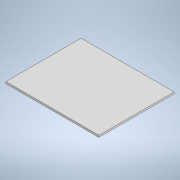
# Autodesk Inventor part: False_Bottom
Saved by Autodesk Inventor 2020 (Build 240168000, 168)
## iProperties
Created: 2021-12-09
Part Number: False_Bottom
Material: Generic
Document SubType Name: Modeling
Designer: danie
Density: 1 g/cm^3
Appearance: Default
Author: danie
Autodesk Inventor part; units mm, degrees
ref_plane "YZ Plane" through (0, 0, 0) normal (1, 0, 0) x (0, 1, 0)
ref_plane "XZ Plane" through (0, 0, 0) normal (0, 1, 0) x (-1, 0, 0)
ref_plane "XY Plane" through (0, 0, 0) normal (0, 0, 1) x (1, 0, 0)
sketch "Sketch1" plane through (0, 0, 0) normal (0, 1, 0) x (-1, 0, 0)
  line L0 (0, 0) -> (-155.575, 0)
  line L1 (-155.575, 0) -> (-155.575, 125.73)
  line L2 (-155.575, 125.73) -> (0, 125.73)
  line L3 (0, 125.73) -> (0, 0)
  dimension "d0" = 155.575
  dimension "d1" = 125.73
  constraints: 8 end point, 2 parallel, 1 horizontal, 1 perpendicular
  measures "d0" distance of L1.end L2.end
  measures "d1" distance of L0.end L1.end
extrude "Extrusion1" add sketch "Sketch1" along normal blind 3.175
sketch "Sketch2" plane through (0, 0, 0) normal (0, -1, 0) x (1, 0, 0)
  line L0 (155.575, 0) -> (0, 0) construction
  line L1 (0, 0) -> (12.7, 0) construction
  line L2 (0, 125.73) -> (155.575, 125.73) construction
  line L3 (12.7, 0) -> (15.875, 0) construction
  line L4 (15.875, 0) -> (15.875, 125.73) construction
  line L5 (15.875, 125.73) -> (12.7, 125.73) construction
  line L6 (12.7, 125.73) -> (12.7, 0) construction
  line L7 (15.875, 0) -> (92.075, 0) construction
  line L8 (23.8468, 0) -> (23.8468, 8.89) construction
  line L9 (23.8468, 125.73) -> (23.8468, 116.84) construction
  line L10 (23.8468, 8.89) -> (15.875, 8.89) construction
  line L11 (23.8468, 116.84) -> (15.875, 116.84) construction
  line L12 (92.075, 0) -> (92.075, 125.73) construction
  line L13 (23.8468, 116.84) -> (92.075, 116.84) construction
  line L14 (23.8468, 8.89) -> (92.075, 8.89) construction
  line L15 (15.875, 8.89) -> (12.7, 8.89)
  line L16 (12.7, 8.89) -> (12.7, 116.84)
  line L17 (12.7, 116.84) -> (15.875, 116.84)
  line L18 (15.875, 116.84) -> (15.875, 8.89)
  line L19 (92.075, 8.89) -> (95.25, 8.89)
  line L20 (95.25, 8.89) -> (95.25, 116.84)
  line L21 (95.25, 116.84) -> (92.075, 116.84)
  line L22 (92.075, 116.84) -> (92.075, 8.89)
  dimension "d4" = 12.7
  dimension "d5" = 3.175
  dimension "d6" = 76.2
  dimension "d11" = 8.89
  dimension "d12" = 8.89
  dimension "d13" = 3.175
  dimension "d14" = 107.95
  constraints: 42 end point, 11 point on line, 8 perpendicular, 7 parallel, 3 horizontal, 1 vertical
  measures "d4" distance of L0.end L1.end
  measures "d5" distance of L5.end L4.end
  measures "d6" distance of L3.end L7.end
  measures "d11" distance of L8.start L8.end
  measures "d12" distance of L9.start L9.end
  measures "d13" distance of L21.end L20.end
  measures "d14" distance of L20.end L19.end
extrude "Extrusion2" add sketch "Sketch2" along normal blind 6.35
body "Solid1"
